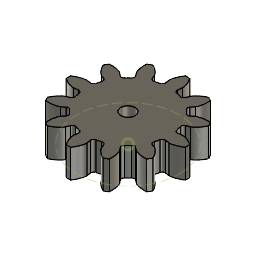
Gear and Slider (Autodesk Fusion 360 archive; units mm, degrees)
design "Spur Gear 12 teeth"
description: Spur Gear; Module: 3.0; Num Teeth: 12; Pressure Angle: 20.0; Backlash: 0.50 mm
Autodesk Fusion 360 part; units mm, degrees
sketch "Base Circle" plane through (0, 0, 0) normal (0, 0, 1) x (1, 0, 0)
  circle A0 centre (0, 0) radius 14.529
  circle A1 centre (0, 0) radius 2.5
extrude "Extrude1" add sketch "Base Circle" along normal blind 10
sketch "Gear Tooth" plane through (0, 0, 0) normal (0, 0, 1) x (1, 0, 0)
  spline S0 degree 5 poles (16.7517, -2.3412) (16.7637, -2.3429) (16.7879, -2.3459) (16.8242, -2.3492) (16.8728, -2.3514) (16.9338, -2.3511) (16.995, -2.3487) (17.0562, -2.3449) (17.1175, -2.3405) (17.1789, -2.3355) (17.2403, -2.33) (17.3018, -2.3238) (17.3632, -2.3167) (17.4248, -2.3085) (17.4863, -2.2992) (17.5479, -2.2889) (17.6095, -2.2778) (17.6711, -2.266) (17.7327, -2.2535) (17.7943, -2.2405) (17.8559, -2.2269) (17.9175, -2.2126) (17.979, -2.1977) (18.0406, -2.1821) (18.1021, -2.1658) (18.1637, -2.1489) (18.2251, -2.1313) (18.2866, -2.1132) (18.348, -2.0945) (18.4094, -2.0753) (18.4708, -2.0555) (18.5321, -2.0351) (18.5934, -2.0142) (18.6546, -1.9928) (18.7158, -1.9708) (18.7769, -1.9483) (18.838, -1.9253) (18.8991, -1.9017) (18.96, -1.8776) (19.0209, -1.8531) (19.0818, -1.828) (19.1426, -1.8024) (19.2033, -1.7764) (19.264, -1.7498) (19.3246, -1.7228) (19.3851, -1.6953) (19.4455, -1.6674) (19.5059, -1.6389) (19.5662, -1.61) (19.6264, -1.5807) (19.6865, -1.5508) (19.7466, -1.5206) (19.8065, -1.4898) (19.8664, -1.4587) (19.9262, -1.4271) (19.9859, -1.395) (20.0455, -1.3625) (20.105, -1.3296) (20.1645, -1.2962) (20.2238, -1.2624) (20.283, -1.2282) (20.3421, -1.1936) (20.4011, -1.1585) (20.4601, -1.1231) (20.5189, -1.0872) (20.5776, -1.0509) (20.6362, -1.0142) (20.6946, -0.977) (20.753, -0.9395) (20.8113, -0.9016) (20.8694, -0.8633) (20.9158, -0.8323) (20.9506, -0.8089) (20.9737, -0.7932) (20.9853, -0.7853) knots 0 0 0 0 0 0 0.01428571 0.02857143 0.04285714 0.05714286 0.07142857 0.08571429 0.1 0.11428571 0.12857143 0.14285714 0.15714286 0.17142857 0.18571429 0.2 0.21428571 0.22857143 0.24285714 0.25714286 0.27142857 0.28571429 0.3 0.31428571 0.32857143 0.34285714 0.35714286 0.37142857 0.38571429 0.4 0.41428571 0.42857143 0.44285714 0.45714286 0.47142857 0.48571429 0.5 0.51428571 0.52857143 0.54285714 0.55714286 0.57142857 0.58571429 0.6 0.61428571 0.62857143 0.64285714 0.65714286 0.67142857 0.68571429 0.7 0.71428571 0.72857143 0.74285714 0.75714286 0.77142857 0.78571429 0.8 0.81428571 0.82857143 0.84285714 0.85714286 0.87142857 0.88571429 0.9 0.91428571 0.92857143 0.94285714 0.95714286 0.97142857 0.98571429 1 1 1 1 1 1
  spline S1 degree 5 poles (16.7517, 2.3412) (16.7637, 2.3429) (16.7879, 2.3459) (16.8242, 2.3492) (16.8728, 2.3514) (16.9338, 2.3511) (16.995, 2.3487) (17.0562, 2.3449) (17.1175, 2.3405) (17.1789, 2.3355) (17.2403, 2.33) (17.3018, 2.3238) (17.3632, 2.3167) (17.4248, 2.3085) (17.4863, 2.2992) (17.5479, 2.2889) (17.6095, 2.2778) (17.6711, 2.266) (17.7327, 2.2535) (17.7943, 2.2405) (17.8559, 2.2269) (17.9175, 2.2126) (17.979, 2.1977) (18.0406, 2.1821) (18.1021, 2.1658) (18.1637, 2.1489) (18.2251, 2.1313) (18.2866, 2.1132) (18.348, 2.0945) (18.4094, 2.0753) (18.4708, 2.0555) (18.5321, 2.0351) (18.5934, 2.0142) (18.6546, 1.9928) (18.7158, 1.9708) (18.7769, 1.9483) (18.838, 1.9253) (18.8991, 1.9017) (18.96, 1.8776) (19.0209, 1.8531) (19.0818, 1.828) (19.1426, 1.8024) (19.2033, 1.7764) (19.264, 1.7498) (19.3246, 1.7228) (19.3851, 1.6953) (19.4455, 1.6674) (19.5059, 1.6389) (19.5662, 1.61) (19.6264, 1.5807) (19.6865, 1.5508) (19.7466, 1.5206) (19.8065, 1.4898) (19.8664, 1.4587) (19.9262, 1.4271) (19.9859, 1.395) (20.0455, 1.3625) (20.105, 1.3296) (20.1645, 1.2962) (20.2238, 1.2624) (20.283, 1.2282) (20.3421, 1.1936) (20.4011, 1.1585) (20.4601, 1.1231) (20.5189, 1.0872) (20.5776, 1.0509) (20.6362, 1.0142) (20.6946, 0.977) (20.753, 0.9395) (20.8113, 0.9016) (20.8694, 0.8633) (20.9158, 0.8323) (20.9506, 0.8089) (20.9737, 0.7932) (20.9853, 0.7853) knots 0 0 0 0 0 0 0.01428571 0.02857143 0.04285714 0.05714286 0.07142857 0.08571429 0.1 0.11428571 0.12857143 0.14285714 0.15714286 0.17142857 0.18571429 0.2 0.21428571 0.22857143 0.24285714 0.25714286 0.27142857 0.28571429 0.3 0.31428571 0.32857143 0.34285714 0.35714286 0.37142857 0.38571429 0.4 0.41428571 0.42857143 0.44285714 0.45714286 0.47142857 0.48571429 0.5 0.51428571 0.52857143 0.54285714 0.55714286 0.57142857 0.58571429 0.6 0.61428571 0.62857143 0.64285714 0.65714286 0.67142857 0.68571429 0.7 0.71428571 0.72857143 0.74285714 0.75714286 0.77142857 0.78571429 0.8 0.81428571 0.82857143 0.84285714 0.85714286 0.87142857 0.88571429 0.9 0.91428571 0.92857143 0.94285714 0.95714286 0.97142857 0.98571429 1 1 1 1 1 1
  arc A0 (20.9853, -0.7853) -> (20.9853, 0.7853) centre (0, 0) ccw
  line L0 (14.3792, -2.0096) -> (16.7517, -2.3412)
  line L1 (14.3792, 2.0096) -> (16.7517, 2.3412)
  line L2 (14.3792, -2.0096) -> (14.3792, 2.0096)
  point P0 (17.0457, -2.3455)
  point P1 (17.3438, -2.3188)
  point P2 (17.6444, -2.271)
  point P3 (17.9468, -2.2054)
  point P4 (18.2504, -2.1238)
  point P5 (18.555, -2.0273)
  point P6 (18.8601, -1.9167)
  point P7 (19.1654, -1.7926)
  point P8 (19.4706, -1.6555)
  point P9 (19.7755, -1.5057)
  point P10 (20.0796, -1.3436)
  point P11 (20.3828, -1.1693)
  point P12 (20.6848, -0.9832)
  point P13 (17.0457, 2.3455)
  point P14 (17.3438, 2.3188)
  point P15 (17.6444, 2.271)
  point P16 (17.9468, 2.2054)
  point P17 (18.2504, 2.1238)
  point P18 (18.555, 2.0273)
  point P19 (18.8601, 1.9167)
  point P20 (19.1654, 1.7926)
  point P21 (19.4706, 1.6555)
  point P22 (19.7755, 1.5057)
  point P23 (20.0796, 1.3436)
  point P24 (20.3828, 1.1693)
  point P25 (20.6848, 0.9832)
extrude "Extrude2" add sketch "Gear Tooth" along normal blind 10
fillet "Fillet1" radius 1 2 edges at (14.3892, -2.011, 5) (14.3892, 2.011, 5)
pattern_circular "C-Pattern1" count 12 over 360 about axis through (0, 0, 0) along (0, 0, 1) of "Extrude2", "Fillet1"
sketch "Diametrial Pitch Circle" plane through (0, 0, 0) normal (0, 0, 1) x (1, 0, 0)
  circle A0 centre (0, 0) radius 18 construction
